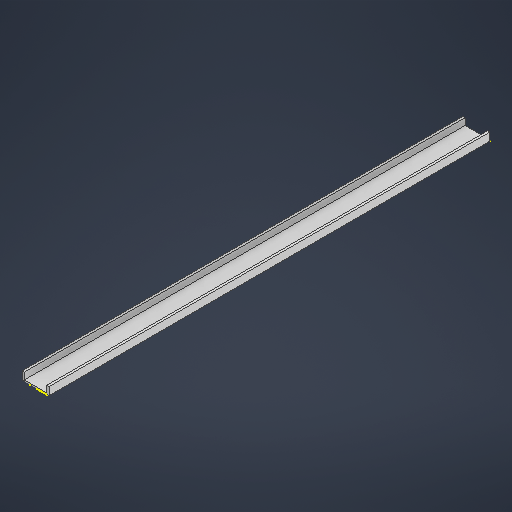
# Autodesk Inventor part: 3 часть направляшки
Saved by Autodesk Inventor 2025 (Build 290162000, 162)
## iProperties
Created: 2024-11-23
Part Number: 3 часть направляшки
Material: Типовые
Document SubType Name: Modeling
Designer: Phantom
Density: 1 g/cm^3
Appearance: По умолчанию
Author: Phantom
Autodesk Inventor part; units mm, degrees
ref_plane "YZ Plane" through (0, 0, 0) normal (1, 0, 0) x (0, 1, 0)
ref_plane "XZ Plane" through (0, 0, 0) normal (0, 1, 0) x (-1, 0, 0)
ref_plane "XY Plane" through (0, 0, 0) normal (0, 0, 1) x (1, 0, 0)
sketch "Эскиз1" plane through (0, 0, 0) normal (0, 0, 1) x (1, 0, 0)
  line L0 (0, 0) -> (24, 0)
  line L1 (24, 0) -> (24, 7)
  line L2 (24, 7) -> (0, 7)
  line L3 (0, 7) -> (0, 0)
  line L4 (0, 1) -> (24, 1)
  line L5 (2, 7) -> (2, 0)
  line L6 (22, 7) -> (22, 0)
  point P0 (0, 3.5)
  point P1 (12, 0)
  point P2 (2, 1)
  point P3 (22, 1)
  dimension "d0" = 24
  dimension "d1" = 7
  dimension "d2" = 2
  dimension "d3" = 2
  dimension "d4" = 1
  constraints: 14 end point, 4 perpendicular, 4 point on line, 2 midpoint, 2 parallel, 1 horizontal
  measures "d0" distance of L2.end L1.end
  measures "d1" distance of L1.end L0.end
  measures "d2" distance from line of point (0, 3.5) L5
  measures "d3" distance between parallel lines of L1 L6
  measures "d4" distance from line of point (12, 0) L4
extrude "Выдавливание1" add sketch "Эскиз1" along normal blind 390 contours L3 L4 L5 L0 | L5 L4 L6 L0 | L3 L2 L5 L4 | L6 L4 L1 L0 | L6 L2 L1 L4
sketch "Эскиз2" plane through (0, 0, 0) normal (0, -1, 0) x (1, 0, 0)
  line L0 (0, 0) -> (24, 0) projected
sketch "Эскиз3" plane through (0, 0, 0) normal (0, -1, 0) x (1, 0, 0)
  line L0 (22, 0) -> (2, 0) projected
  line L1 (12, 0) -> (12, 390)
  line L2 (22, 390) -> (2, 390) projected
  point P0 (0, 0)
  constraints: 2 end point, 2 midpoint
